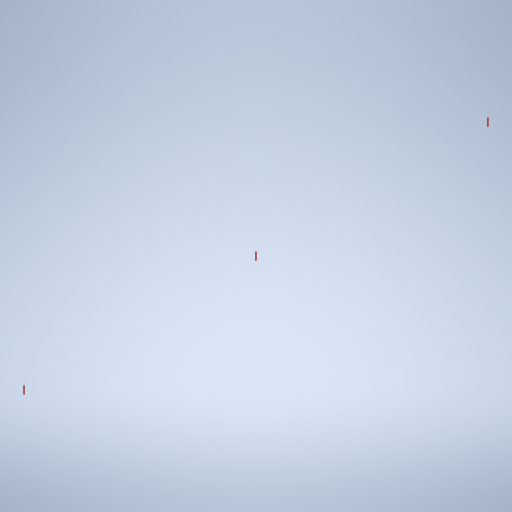
# Autodesk Inventor part: Confirmat Joint1200
Saved by Autodesk Inventor 2024 (Build 280153000, 153)
## iProperties
RuleStatus: InUse
Created: 2023-01-09
Part Number: Confirmat Joint1200
Material: Generic
Document SubType Name: Modeling
Designer: sauliusd
Density: 1 g/cm^3
Appearance: Default
AfterAnyUserParamChange0: ComponenetsArrayParams
AfterAnyParamChange0: ComponenetsArrayParams
Author: sauliusd
Autodesk Inventor part; units mm, degrees
ref_plane "YZ Plane" through (0, 0, 0) normal (1, 0, 0) x (0, 1, 0)
ref_plane "XZ Plane" through (0, 0, 0) normal (0, 1, 0) x (-1, 0, 0)
ref_plane "XY Plane" through (0, 0, 0) normal (0, 0, 1) x (1, 0, 0)
sketch "Sketch1" plane through (0, 0, 0) normal (0, 0, 1) x (1, 0, 0)
  line L0 (-357, -9) -> (357, -9)
  line L1 (357, -9) -> (357, 9)
  line L2 (357, 9) -> (-357, 9)
  line L3 (-357, 9) -> (-357, -9)
  line L4 (-357, -9) -> (357, 9) construction
  line L5 (357, -9) -> (-357, 9) construction
  point P0 (0, 0)
  dimension "d0" = 714
  dimension "d1" = 18
  constraints: 12 end point, 2 midpoint, 2 parallel, 1 horizontal, 1 perpendicular
  measures "d0" distance of L2.end L1.end
  measures "d1" distance of L0.end L1.end
sketch "Sketch2" plane through (0, 0, 0) normal (0, 0, 1) x (1, 0, 0)
  circle A0 centre (288, 0) radius 0.5
  line L0 (357, 9) -> (-357, 9) projected
  line L1 (-357, -9) -> (357, -9) projected
  line L2 (0, -12.6) -> (0, 12.6) projected
  line L3 (357, -9) -> (357, 9) projected
  point P0 (0, 0)
  point P1 (357, 0)
  dimension "d4" = 1
  dimension "d26" = 69
  constraints: 1 centre point, 1 horizontal alignment, 1 midpoint
  measures "d4" diameter of A0
  measures "d26" distance from line of L3 A0.centre
extrude "Extrusion1" add sketch "Sketch2" along normal blind 10 contours A0
pattern_linear "Confirmat Array" count 3 spacing 288 along (-1, 0, 0) of "Extrusion1"
equation "\"d26\" = X_Coord"
equation "\"d9\" = Step"
equation "\"d0\" = ContactPatchWidth"
equation "\"d1\" = ContactPatchHeight"
equation "\"ContactPatchWidth\" = 714"
equation "\"ContactPatchHeight\" = 18"
equation "\"PlacingStep\" = 32"
equation "\"PlacingWidth\" = -MinDistFromSide1 + ContactPatchWidth - MinDistFromSide2"
equation "\"PlacingWithByStep\" = 576"
equation "\"X_Coord\" = 69"
equation "\"Step\" = 288"
equation "\"Y_Coord\" = 9.5"
equation "\"CenterX_Coord\" = MinDistFromSide1 + 0.5 * PlacingWidth"
equation "\"MaxDistBetweenByStep\" = 192"
equation "\"DistBetween\" = 297"
equation "\"MinDistFromSide1\" = 60"
equation "\"MinDistFromSide2\" = 60"
